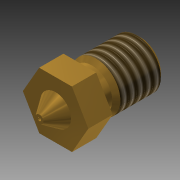
# Autodesk Inventor part: e3d_v6_nozzle
Saved by Autodesk Inventor 2013 (Build 170138000, 138)
## iProperties
Created: 2015-02-20
Part Number: e3d_v6_nozzle
Material: 一般
Document SubType Name: Modeling
Designer: Noa Izumi
Density: 1 g/cm^3
Author: Noa Izumi
Autodesk Inventor part; units mm, degrees
ref_plane "YZ Plane" through (0, 0, 0) normal (1, 0, 0) x (0, 1, 0)
ref_plane "XZ Plane" through (0, 0, 0) normal (0, 1, 0) x (-1, 0, 0)
ref_plane "XY Plane" through (0, 0, 0) normal (0, 0, 1) x (1, 0, 0)
sketch "草圖1" plane through (0, 0, 0) normal (0, 1, 0) x (-1, 0, 0)
  line L0 (2.0138, -3.504) -> (-2.0277, -3.496)
  line L1 (-2.0277, -3.496) -> (-4.0414, 0.008)
  line L2 (-4.0414, 0.008) -> (-2.0138, 3.504)
  line L3 (-2.0138, 3.504) -> (2.0277, 3.496)
  line L4 (2.0277, 3.496) -> (4.0414, -0.008)
  line L5 (4.0414, -0.008) -> (2.0138, -3.504)
  point P0 (0, 0)
  point P1 (0, 0)
  dimension "d0" = 7
  constraints: 12 end point, 1 coincident, 13 other
  measures "d0" distance between parallel lines of L0 L3
extrude "擠出1" add sketch "草圖1" along normal blind 3
sketch "草圖2" plane through (0, 3, 0) normal (0, 1, 0) x (1, 0, 0)
  circle A0 centre (0, 0) radius 2.5
  dimension "d3" = 5
  constraints: 1 centre point, 1 coincident
  measures "d3" diameter of A0
extrude "擠出2" add sketch "草圖2" along normal blind 1.5
sketch "草圖3" plane through (0, 4.5, 0) normal (0, 1, 0) x (1, 0, 0)
  circle A0 centre (0, 0) radius 2.5 projected
  circle A1 centre (0, 0) radius 3
  dimension "d7" = 6
  constraints: 1 centre point, 1 coincident
  measures "d7" diameter of A1
extrude "擠出3" add sketch "草圖3" along normal blind 6 contours A0 | A1
sketch "草圖4" plane through (0, 0, 0) normal (0, -1, 0) x (1, 0, 0)
  circle A0 centre (0, 0) radius 1.9
  dimension "d11" = 3.8
  constraints: 1 centre point, 1 coincident
  measures "d11" diameter of A0
extrude "擠出4" add sketch "草圖4" along normal blind 2 draft -35
sketch "草圖5" plane through (0, 10.5, 0) normal (0, 1, 0) x (1, 0, 0)
  circle A0 centre (0, 0) radius 3 projected
  constraints: 1 coincident
hole "孔1" at (0, 10.5, 0) direction (0, -1, 0) diameter 2 depth 10.5 tip angle 118
chamfer "倒角1" distance 0.5 angle 45 3 edges at (-3, 4.5, 0) (-3, 10.5, 0) (0, 10.5, -1)
thread "螺紋1" size "M6x1" class "6g" standard "ANSI Metric M Profile" full length
sketch "草圖6" plane through (0, -2, 0) normal (0, -1, 0) x (1, 0, 0)
  circle A0 centre (0, 0) radius 0.4996 projected
  constraints: 1 coincident
hole "孔2" at (0, -2, 0) direction (0, 1, 0) diameter 0.4 end through all
sketch "草圖7" plane through (0, 10.5, 0) normal (0, 1, 0) x (1, 0, 0)
  circle A0 centre (0, 0) radius 1.5 projected
  constraints: 1 coincident
hole "孔3" at (0, 10.5, 0) direction (0, -1, 0) diameter 1.5 depth 11.5 tip angle 118
